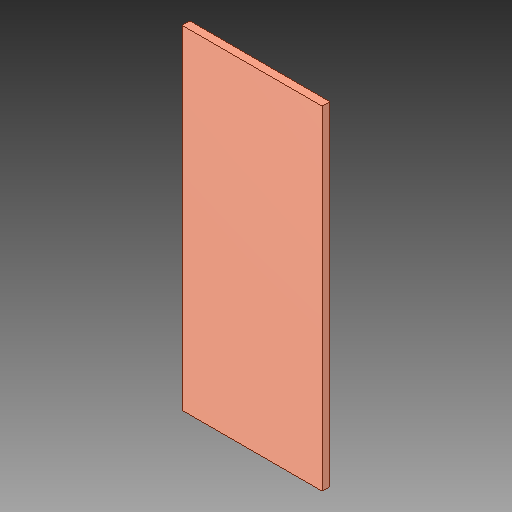
# Autodesk Inventor part: E01-ML01DP5
Saved by Autodesk Inventor 2019 (Build 230136000, 136)
## iProperties
Created: 2019-10-02
Part Number: E01-ML01DP5
Material: Generic
Document SubType Name: Modeling
Designer: rybit
Density: 1 g/cm^3
Appearance: E01-ML01DP5, E01-ML01DP5
Author: rybit
Autodesk Inventor part; units mm, degrees
ref_plane "YZ Plane" through (0, 0, 0) normal (1, 0, 0) x (0, 1, 0)
ref_plane "XZ Plane" through (0, 0, 0) normal (0, 1, 0) x (-1, 0, 0)
ref_plane "XY Plane" through (0, 0, 0) normal (0, 0, 1) x (1, 0, 0)
sketch "E01-ML01DP5, E01-ML01DP5_23" plane through (0, 0, 0) normal (0, 0, 1) x (1, 0, 0)
  line L0 (-0.1016, 0.1016) -> (18, 0.1016)
  line L1 (18, 0.1016) -> (18, -43)
  line L2 (18, -43) -> (-0.1016, -43)
  line L3 (-0.1016, -43) -> (-0.1016, 0.1016)
  constraints: 8 end point
extrude "Extrusion1" add sketch "E01-ML01DP5, E01-ML01DP5_23" along normal blind 1
body "Solid1"
